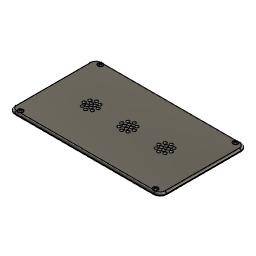
_Raspi7inch_LidBig.b8c6004f-4b55-48d0-a08e-654ef1e60da1 (Autodesk Fusion 360 design; units mm, degrees)
Autodesk Fusion 360 part; units mm, degrees
sketch "Sketch1" plane through (0, 0, 0) normal (0, 0, 1) x (1, 0, 0)
  line L0 (8, 0) -> (185, 0)
  line L1 (193, 8) -> (193, 103)
  line L2 (185, 111) -> (8, 111)
  line L3 (0, 103) -> (0, 8)
  arc A0 (8, 111) -> (0, 103) centre (8, 103) ccw
  arc A1 (193, 103) -> (185, 111) centre (185, 103) ccw
  arc A2 (185, 0) -> (193, 8) centre (185, 8) ccw
  arc A3 (0, 8) -> (8, 0) centre (8, 8) ccw
  point P0 (193, 0)
  point P1 (0, 111)
  dimension "d1" = 193
  dimension "d2" = 111
  dimension "d3" = 8
  dimension "d4" = 8
  dimension "d5" = 8
  dimension "d6" = 8
  constraint horizontal L0
  constraint vertical L1
  constraint horizontal L2
  constraint vertical L3
  constraint coincident P1 L2
  constraint coincident P1 L3
  constraint tangent L2 A0
  constraint tangent L3 A0
  constraint tangent L1 A1
  constraint tangent L2 A1
  constraint coincident P0 L0
  constraint coincident P0 L1
  constraint tangent L0 A2
  constraint tangent L1 A2
  constraint coincident origin L0
  constraint coincident origin L3
  constraint tangent L0 A3
  constraint tangent L3 A3
  measures "d1" distance of origin P0
  measures "d2" distance of origin P1
  measures "d3" radius of A0
  measures "d4" radius of A1
  measures "d5" radius of A2
  measures "d6" radius of A3
extrude "Extrude1" add sketch "Sketch1" along normal blind 3
fillet "Fillet1" radius 2 8 edges at (193, 55.5, 3) (190.6569, 108.6569, 3) (96.5, 111, 3) (2.3431, 108.6569, 3) (0, 55.5, 3) (2.3431, 2.3431, 3) (96.5, 0, 3) (190.6569, 2.3431, 3)
sketch "Sketch2" plane through (0, 0, 3) normal (0, 0, 1) x (-1, 0, 0)
  line L0 (-191, -8) -> (-191, -103)
  arc A0 (-191, -103) -> (-185, -109) centre (-185, -103) ccw
  line L1 (-185, -109) -> (-8, -109)
  arc A1 (-8, -109) -> (-2, -103) centre (-8, -103) ccw
  line L2 (-2, -103) -> (-2, -8)
  arc A2 (-2, -8) -> (-8, -2) centre (-8, -8) ccw
  line L3 (-8, -2) -> (-185, -2)
  arc A3 (-185, -2) -> (-191, -8) centre (-185, -8) ccw
  line L4 (-8, -109) -> (-13, -109)
  line L5 (-13, -109) -> (-13, -104)
  line L6 (-13, -104) -> (-8, -104)
  line L7 (-8, -104) -> (-8, -109)
  circle A4 centre (-10.5, -106.5) radius 1.6
  line L8 (-185, -109) -> (-180, -109)
  line L9 (-180, -109) -> (-180, -104)
  line L10 (-180, -104) -> (-185, -104)
  line L11 (-185, -104) -> (-185, -109)
  circle A5 centre (-182.5, -106.5) radius 1.6
  line L12 (-185, -2) -> (-180, -2)
  line L13 (-180, -2) -> (-180, -7)
  line L14 (-180, -7) -> (-185, -7)
  line L15 (-185, -7) -> (-185, -2)
  circle A6 centre (-182.5, -4.5) radius 1.6
  line L16 (-8, -2) -> (-13, -2)
  line L17 (-13, -2) -> (-13, -7)
  line L18 (-13, -7) -> (-8, -7)
  line L19 (-8, -7) -> (-8, -2)
  circle A7 centre (-10.5, -4.5) radius 1.6
  point P0 (-10.5, -106.5)
  dimension "d11" = 5
  dimension "d12" = 5
  dimension "d13" = 3.2
  dimension "d14" = 5
  dimension "d15" = 5
  dimension "d16" = 3.2
  dimension "d17" = 5
  dimension "d18" = 5
  dimension "d19" = 3.2
  dimension "d20" = 5
  dimension "d21" = 5
  dimension "d22" = 3.2
  constraint horizontal L4
  constraint vertical L5
  constraint horizontal L6
  constraint vertical L7
  constraint coincident L1.end A1.start
  constraint coincident P0 A4.centre
  constraint horizontal L8
  constraint vertical L9
  constraint horizontal L10
  constraint vertical L11
  constraint coincident A0.end L1.start
  constraint horizontal L12
  constraint vertical L13
  constraint horizontal L14
  constraint vertical L15
  constraint coincident L3.end A3.start
  constraint horizontal L16
  constraint vertical L17
  constraint horizontal L18
  constraint vertical L19
  constraint coincident A2.end L3.start
  measures "d11" distance of L1.end L4.end
  measures "d12" distance of L1.end L6.end
  measures "d13" diameter of A4
  measures "d14" distance of A0.end L8.end
  measures "d15" distance of A0.end L10.end
  measures "d16" diameter of A5
  measures "d17" distance of L3.end L12.end
  measures "d18" distance of L3.end L14.end
  measures "d19" diameter of A6
  measures "d20" distance of A2.end L16.end
  measures "d21" distance of A2.end L18.end
  measures "d22" diameter of A7
hole "Hole1" at (10.5, 4.5, 3) at (10.5, 106.5, 3) at (182.5, 106.5, 3) at (182.5, 4.5, 3) direction (0, 0, -1) diameter 3.2 depth 7 tip angle 180
sketch "Sketch3" plane through (0, 0, 3) normal (0, 0, 1) x (-1, 0, 0)
  circle A0 centre (-182.5, -106.5) radius 1.6
  circle A1 centre (-10.5, -4.5) radius 1.6
  circle A2 centre (-10.5, -106.5) radius 1.6
  circle A3 centre (-182.5, -4.5) radius 1.6
  line L0 (-191, -8) -> (-191, -103)
  arc A4 (-191, -103) -> (-185, -109) centre (-185, -103) ccw
  line L1 (-185, -109) -> (-8, -109)
  arc A5 (-8, -109) -> (-2, -103) centre (-8, -103) ccw
  line L2 (-2, -103) -> (-2, -8)
  arc A6 (-2, -8) -> (-8, -2) centre (-8, -8) ccw
  line L3 (-8, -2) -> (-185, -2)
  arc A7 (-185, -2) -> (-191, -8) centre (-185, -8) ccw
  circle A8 centre (-10.5, -106.5) radius 3.2
  circle A9 centre (-182.5, -106.5) radius 3.2
  circle A10 centre (-182.5, -4.5) radius 3.2
  circle A11 centre (-10.5, -4.5) radius 3.2
  dimension "d26" = 6.4
  dimension "d27" = 6.4
  dimension "d28" = 6.4
  dimension "d29" = 6.4
  constraint concentric A2 A8
  constraint concentric A0 A9
  constraint concentric A3 A10
  constraint concentric A1 A11
  measures "d26" diameter of A8
  measures "d27" diameter of A9
  measures "d28" diameter of A10
  measures "d29" diameter of A11
hole "Hole2" at (182.5, 4.5, 3) at (10.5, 4.5, 3) at (182.5, 106.5, 3) at (10.5, 106.5, 3) direction (0, 0, -1) diameter 6.4 depth 0.854 tip angle 180
sketch "Sketch4" plane through (0, 0, 3) normal (0, 0, 1) x (-1, 0, 0)
  arc A0 (-180.5025, -109) -> (-184.4975, -109) centre (-182.5, -106.5) ccw
  line L0 (-180.5025, -109) -> (-12.4975, -109)
  arc A1 (-8.5025, -109) -> (-12.4975, -109) centre (-10.5, -106.5) ccw
  line L1 (-8.5025, -109) -> (-8, -109)
  arc A2 (-8, -109) -> (-2, -103) centre (-8, -103) ccw
  line L2 (-2, -103) -> (-2, -8)
  arc A3 (-2, -8) -> (-8, -2) centre (-8, -8) ccw
  line L3 (-8, -2) -> (-8.5025, -2)
  arc A4 (-12.4975, -2) -> (-8.5025, -2) centre (-10.5, -4.5) ccw
  line L4 (-12.4975, -2) -> (-180.5025, -2)
  arc A5 (-184.4975, -2) -> (-180.5025, -2) centre (-182.5, -4.5) ccw
  line L5 (-184.4975, -2) -> (-185, -2)
  arc A6 (-185, -2) -> (-191, -8) centre (-185, -8) ccw
  line L6 (-191, -8) -> (-191, -103)
  arc A7 (-191, -103) -> (-185, -109) centre (-185, -103) ccw
  line L7 (-185, -109) -> (-184.4975, -109)
  circle A8 centre (-41.5919, -54.4399) radius 2
  circle A9 centre (-44.664, -49.1434) radius 2
  circle A10 centre (-50.5814, -47.5705) radius 2
  circle A11 centre (-55.8779, -50.6426) radius 2
  circle A12 centre (-57.4508, -56.5601) radius 2
  circle A13 centre (-54.3787, -61.8566) radius 2
  circle A14 centre (-48.4612, -63.4295) radius 2
  circle A15 centre (-43.1648, -60.3574) radius 2
  circle A16 centre (-46.9732, -53.1006) radius 2
  circle A17 centre (-51.9207, -52.9519) radius 2
  circle A18 centre (-52.0695, -57.8994) radius 2
  circle A19 centre (-47.122, -58.0481) radius 2
  circle A20 centre (-95.1603, -58.7335) radius 2
  circle A21 centre (-96.5061, -47.5) radius 2
  circle A22 centre (-102.1612, -49.8474) radius 2
  circle A23 centre (-96.4939, -63.5) radius 2
  circle A24 centre (-104.5, -55.5061) radius 2
  circle A25 centre (-93.2665, -54.1603) radius 2
  circle A26 centre (-99.7335, -56.8397) radius 2
  circle A27 centre (-90.8474, -49.8388) radius 2
  circle A28 centre (-90.8388, -61.1526) radius 2
  circle A29 centre (-97.8397, -52.2665) radius 2
  circle A30 centre (-102.1526, -61.1612) radius 2
  circle A31 centre (-88.5, -55.4939) radius 2
  circle A32 centre (-147.0416, -56.8385) radius 2
  circle A33 centre (-151.8076, -55.479) radius 2
  circle A34 centre (-142.4691, -58.734) radius 2
  circle A35 centre (-138.1359, -49.858) radius 2
  circle A36 centre (-138.1656, -61.1717) radius 2
  circle A37 centre (-143.8286, -63.5) radius 2
  circle A38 centre (-143.7866, -47.5) radius 2
  circle A39 centre (-149.4793, -61.142) radius 2
  circle A40 centre (-149.4496, -49.8283) radius 2
  circle A41 centre (-145.1461, -52.266) radius 2
  circle A42 centre (-135.8076, -55.521) radius 2
  circle A43 centre (-140.5736, -54.1615) radius 2
  point P0 (-49.5213, -55.5)
  point P1 (-96.5, -55.5)
  point P2 (-143.8076, -55.5)
  dimension "d33" = 8
  dimension "d34" = 4
  dimension "d37" = 360
  dimension "d40" = 3.5
  dimension "d41" = 4
  dimension "d43" = 360
  dimension "d45" = 360
  dimension "d47" = 360
  dimension "d48" = 8
  dimension "d49" = 4
  dimension "d50" = 3.5
  dimension "d51" = 4
  dimension "d55" = 360
  dimension "d57" = 360
  dimension "d58" = 8
  dimension "d59" = 4
  dimension "d60" = 3.5
  dimension "d61" = 4
  measures "d33" distance of P0 A8.centre
  measures "d34" diameter of A8
  measures "d40" distance of P0 A16.centre
  measures "d41" diameter of A16
  measures "d48" distance of P1 A31.centre
  measures "d49" diameter of A31
  measures "d50" distance of P1 A25.centre
  measures "d51" diameter of A25
  measures "d58" distance of P2 A42.centre
  measures "d59" diameter of A42
  measures "d60" distance of P2 A43.centre
  measures "d61" diameter of A43
hole "Hole3" at (52.0695, 57.8994, 3) at (47.122, 58.0481, 3) at (48.4612, 63.4295, 3) at (43.1648, 60.3574, 3) at (41.5919, 54.4399, 3) at (46.9732, 53.1006, 3) at (44.664, 49.1434, 3) at (55.8779, 50.6426, 3) at (51.9207, 52.9519, 3) at (50.5814, 47.5705, 3) at (57.4508, 56.5601, 3) at (54.3787, 61.8566, 3) at (96.4939, 63.5, 3) at (90.8388, 61.1526, 3) at (88.5, 55.4939, 3) at (95.1603, 58.7335, 3) at (93.2665, 54.1603, 3) at (97.8397, 52.2665, 3) at (90.8474, 49.8388, 3) at (96.5061, 47.5, 3) at (102.1612, 49.8474, 3) at (102.1526, 61.1612, 3) at (104.5, 55.5061, 3) at (99.7335, 56.8397, 3) at (142.4691, 58.734, 3) at (138.1656, 61.1717, 3) at (143.8286, 63.5, 3) at (149.4793, 61.142, 3) at (147.0416, 56.8385, 3) at (149.4496, 49.8283, 3) at (145.1461, 52.266, 3) at (151.8076, 55.479, 3) at (143.7866, 47.5, 3) at (138.1359, 49.858, 3) at (140.5736, 54.1615, 3) at (135.8076, 55.521, 3) direction (0, 0, -1) diameter 4 depth 10 tip angle 180
